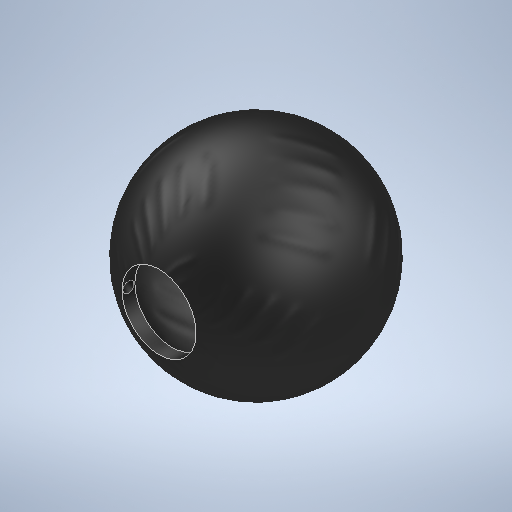
# Autodesk Inventor part: Bola_0002
Saved by Autodesk Inventor 2025.2 (Build 292293000, 293)
## iProperties
Created: 2025-03-26
Part Number: Bola_0002
Material: Generic
Document SubType Name: Modeling
Designer: ishad
Density: 1 g/cm^3
Appearance: Diamond plate - Dark Gray
Author: ishad
Autodesk Inventor part; units mm, degrees
ref_plane "YZ Plane" through (0, 0, 0) normal (1, 0, 0) x (0, 1, 0)
ref_plane "XZ Plane" through (0, 0, 0) normal (0, 1, 0) x (-1, 0, 0)
ref_plane "XY Plane" through (0, 0, 0) normal (0, 0, 1) x (1, 0, 0)
sketch "Sketch1" plane through (0, 0, 0) normal (0, 0, 1) x (1, 0, 0)
  arc A0 (0, -7) -> (0, 7) centre (0, 0) ccw
  arc A1 (0, -6.2) -> (0, 6.2) centre (0, 0) ccw
  line L0 (0, 7) -> (0, 6.2)
  line L1 (0, -6.2) -> (0, -7)
  line L2 (0, -9.8) -> (0, 9.8) projected
  dimension "d4" = 0.8
  dimension "d5" = 7
  constraints: 4 end point, 4 point on circle, 2 centre point, 2 coincident, 2 collinear, 1 vertical
  measures "d4" radial gap between concentric circles of A0 A1
  measures "d5" radius of A0
revolve "Revolution1" add sketch "Sketch1" angle 360 about axis through (0, -10, 0) along (0, -1, 0) contours L1 A1 L0 A0
sketch "Sketch3" plane through (0, 0, 0) normal (0, 0, 1) x (1, 0, 0)
  circle A0 centre (6.6, 0) radius 0.35
  line L0 (0, -0.49) -> (0, 0.49) projected
  point P0 (0, 0)
  point P1 (0, 0)
  dimension "d6" = 0.7
  dimension "d7" = 6.6
  constraints: 1 centre point, 1 coincident, 1 horizontal alignment
  measures "d6" diameter of A0
  measures "d7" distance of point (0, 0) A0.centre
revolve "Revolution2" cut sketch "Sketch3" angle 360 about axis through (0, -10, 0) along (0, -1, 0)
sketch "Sketch4" plane through (0, 0, 0) normal (0, 0, 1) x (1, 0, 0)
  circle A0 centre (0, 0) radius 2.5
  dimension "d13" = 5
  constraints: 1 centre point, 1 coincident
  measures "d13" diameter of A0
extrude "Extrusion1" cut sketch "Sketch4" along normal mid plane 50
body "Solid1"
